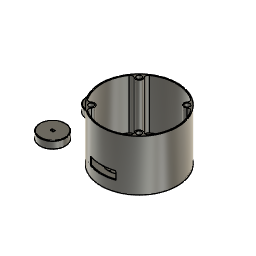
body_bottom_v4 (Autodesk Fusion 360 design; units mm, degrees)
part number: 2025-04-25-05-00-27-819
part number: 2025-04-25-05-02-16-760
part number: 2025-04-28-13-24-04-349
part number: 2025-04-28-13-40-47-946
Autodesk Fusion 360 part; units mm, degrees
sketch "Sketch1" plane through (0, 0, 0) normal (0, 0, 1) x (1, 0, 0) in component "Bottom"
  circle A0 centre (0, 0) radius 75
  dimension "d2" = 150
  constraint coincident A0.centre origin
  measures "d2" diameter of A0
extrude "Extrude1" add sketch "Sketch1" along normal blind 100 makes body 1 in component "Bottom"
shell "Shell1" thickness 2 removed faces 1 at (18.6055, 20.7304, 100) on bodies 1 in component "Bottom"
sketch "Sketch3" plane through (0, 0, 2) normal (0, 0, 1) x (-1, 0, 0) in component "Bottom"
  circle A0 centre (0, 0) radius 73
  circle A1 centre (-67, 0) radius 7
  circle A2 centre (0, 67) radius 7
  circle A3 centre (0, -67) radius 7
  circle A4 centre (67, 0) radius 7
  dimension "d11" = 14
  dimension "d12" = 14
  dimension "d13" = 14
  dimension "d14" = 14
  measures "d11" diameter of A1
  measures "d12" diameter of A2
  measures "d13" diameter of A3
  measures "d14" diameter of A4
extrude "Extrude5" add sketch "Sketch3" along normal blind 98 contours A0 A4 | A0 A2 | A0 A3 | A0 A1 picked at (69.9447, 2.5011) picked at (-0.1343, 68.6633) picked at (-0.1343, -68.6633) picked at (-68.6595, 0) bodies 1 in component "Bottom"
fillet "Fillet1" radius 6 8 edges at (72.903, 3.7623, 51) (72.903, -3.7623, 51) (-3.7623, 72.903, 51) (3.7623, 72.903, 51) (-72.903, -3.7623, 51) (3.7623, -72.903, 51) (-3.7623, -72.903, 51) (-72.903, 3.7623, 51) on bodies 1 in component "Bottom"
sketch "Sketch6" plane through (0, 0, 100) normal (0, 0, 1) x (-1, 0, 0) in component "Bottom"
  arc A0 (71.6259, 14.0974) -> (14.0974, 71.6259) centre (0, 0) ccw
  arc A1 (66.3209, 6.967) -> (71.6259, 14.0974) centre (65.7388, 12.9387) ccw
  arc A2 (66.3209, 6.967) -> (66.3209, -6.967) centre (67, 0) ccw
  arc A3 (71.6259, -14.0974) -> (66.3209, -6.967) centre (65.7388, -12.9387) ccw
  arc A4 (14.0974, -71.6259) -> (71.6259, -14.0974) centre (0, 0) ccw
  arc A5 (6.967, -66.3209) -> (14.0974, -71.6259) centre (12.9387, -65.7388) ccw
  arc A6 (6.967, -66.3209) -> (-6.967, -66.3209) centre (0, -67) ccw
  arc A7 (-14.0974, -71.6259) -> (-6.967, -66.3209) centre (-12.9387, -65.7388) ccw
  arc A8 (-71.6259, -14.0974) -> (-14.0974, -71.6259) centre (0, 0) ccw
  arc A9 (-66.3209, -6.967) -> (-71.6259, -14.0974) centre (-65.7388, -12.9387) ccw
  arc A10 (-66.3209, -6.967) -> (-66.3209, 6.967) centre (-67, 0) ccw
  arc A11 (-71.6259, 14.0974) -> (-66.3209, 6.967) centre (-65.7388, 12.9387) ccw
  arc A12 (-14.0974, 71.6259) -> (-71.6259, 14.0974) centre (0, 0) ccw
  arc A13 (-6.967, 66.3209) -> (-14.0974, 71.6259) centre (-12.9387, 65.7388) ccw
  arc A14 (-6.967, 66.3209) -> (6.967, 66.3209) centre (0, 67) ccw
  arc A15 (14.0974, 71.6259) -> (6.967, 66.3209) centre (12.9387, 65.7388) ccw
  circle A16 centre (0, 0) radius 75
  circle A17 centre (-67, 0) radius 5
  circle A18 centre (0, 67) radius 5
  circle A19 centre (67, 0) radius 5
  circle A20 centre (0, -67) radius 5
  dimension "d26" = 10
  dimension "d27" = 10
  dimension "d28" = 10
  dimension "d29" = 10
  constraint concentric A10 A17
  constraint concentric A14 A18
  constraint concentric A2 A19
  constraint concentric A6 A20
  measures "d26" diameter of A17
  measures "d27" diameter of A18
  measures "d28" diameter of A19
  measures "d29" diameter of A20
extrude "Extrude6" cut sketch "Sketch6" against normal blind 8 contours A17 | A18 | A19 | A20 bodies 1 in component "Bottom"
sketch "Sketch10" plane through (0, 0, 0) normal (0, 1, 0) x (1, 0, 0) in component "Bottom"
  line L0 (0, 100) -> (0, -200)
  constraint vertical L0
ref_plane "WorkPlane1" through (-53.033, 53.033, 0) normal (0.707107, -0.707107, 0) x (0, 0, 1) in component "Bottom"
sketch "Sketch3 (2)" plane through (0, 0, 2) normal (0, 0, 1) x (-1, 0, 0)
  line L0 (-11.65, 45) -> (11.65, 45) construction
  circle A0 centre (-14.35, 45) radius 2.7
  circle A1 centre (14.35, 45) radius 2.7
  line L1 (-14.35, 42.3) -> (-14.35, 19) construction
  line L2 (14.4157, 42.3008) -> (14.4157, 19.0008) construction
  circle A2 centre (-14.35, 16.3) radius 2.7
  circle A3 centre (14.4157, 16.3008) radius 2.7
  arc A4 (-40.6788, 60.6155) -> (-41.9696, 51.8224) centre (-37.3353, 55.6334) ccw
  arc A5 (-51.8224, 41.9696) -> (-41.9696, 51.8224) centre (-47.3762, 47.3762) ccw
  arc A6 (-51.8224, 41.9696) -> (-60.6155, 40.6788) centre (-55.6334, 37.3353) ccw
  arc A7 (-60.6155, 40.6788) -> (-60.6155, -40.6788) centre (0, 0) ccw
  arc A8 (-60.6155, -40.6788) -> (-51.8224, -41.9696) centre (-55.6334, -37.3353) ccw
  arc A9 (-41.9696, -51.8224) -> (-51.8224, -41.9696) centre (-47.3762, -47.3762) ccw
  arc A10 (-41.9696, -51.8224) -> (-40.6788, -60.6155) centre (-37.3353, -55.6334) ccw
  arc A11 (-40.6788, -60.6155) -> (40.6788, -60.6155) centre (0, 0) ccw
  arc A12 (40.6788, -60.6155) -> (41.9696, -51.8224) centre (37.3353, -55.6334) ccw
  arc A13 (51.8224, -41.9696) -> (41.9696, -51.8224) centre (47.3762, -47.3762) ccw
  arc A14 (51.8224, -41.9696) -> (60.6155, -40.6788) centre (55.6334, -37.3353) ccw
  arc A15 (60.6155, -40.6788) -> (60.6155, 40.6788) centre (0, 0) ccw
  arc A16 (60.6155, 40.6788) -> (51.8224, 41.9696) centre (55.6334, 37.3353) ccw
  arc A17 (41.9696, 51.8224) -> (51.8224, 41.9696) centre (47.3762, 47.3762) ccw
  arc A18 (41.9696, 51.8224) -> (40.6788, 60.6155) centre (37.3353, 55.6334) ccw
  arc A19 (40.6788, 60.6155) -> (-40.6788, 60.6155) centre (0, 0) ccw
  dimension "d49" = 23.3
  dimension "d50" = 5.4
  dimension "d51" = 5.4
  dimension "d52" = 23.3
  dimension "d53" = 23.3
  dimension "d54" = 5.4
  dimension "d55" = 5.4
  constraint coincident L0.start A0
  constraint coincident L0.end A1
  constraint coincident A0 L1.start
  constraint coincident A1 L2.start
  constraint coincident L1.end A2
  constraint coincident L2.end A3
  measures "d49" distance of L0.start L0.end
  measures "d50" diameter of A0
  measures "d51" diameter of A1
  measures "d52" distance of L1.start L1.end
  measures "d53" distance of L2.start L2.end
  measures "d54" diameter of A2
  measures "d55" diameter of A3
extrude "Extrude10" cut sketch "Sketch3 (2)" against normal blind 2 contours A0 | A1 | A2 | A3 sketch seen with x (-0.707107, -0.707107, 0) y (0.707107, -0.707107, 0) z (0, 0, 1) at (0, 0, 0) bodies 1 in component "Bottom"
sketch "Sketch4" plane through (0, 0, 2) normal (0, 0, 1) x (-1, 0, 0)
  circle A0 centre (-14.35, 45) radius 2.7
  circle A1 centre (-14.35, 16.3) radius 2.7
  circle A2 centre (14.35, 45) radius 2.7
  circle A3 centre (14.4157, 16.3008) radius 2.7
  arc A4 (-40.6788, 60.6155) -> (-41.9696, 51.8224) centre (-37.3353, 55.6334) ccw
  arc A5 (-51.8224, 41.9696) -> (-41.9696, 51.8224) centre (-47.3762, 47.3762) ccw
  arc A6 (-51.8224, 41.9696) -> (-60.6155, 40.6788) centre (-55.6334, 37.3353) ccw
  arc A7 (-60.6155, 40.6788) -> (-60.6155, -40.6788) centre (0, 0) ccw
  arc A8 (-60.6155, -40.6788) -> (-51.8224, -41.9696) centre (-55.6334, -37.3353) ccw
  arc A9 (-41.9696, -51.8224) -> (-51.8224, -41.9696) centre (-47.3762, -47.3762) ccw
  arc A10 (-41.9696, -51.8224) -> (-40.6788, -60.6155) centre (-37.3353, -55.6334) ccw
  arc A11 (-40.6788, -60.6155) -> (40.6788, -60.6155) centre (0, 0) ccw
  arc A12 (40.6788, -60.6155) -> (41.9696, -51.8224) centre (37.3353, -55.6334) ccw
  arc A13 (51.8224, -41.9696) -> (41.9696, -51.8224) centre (47.3762, -47.3762) ccw
  arc A14 (51.8224, -41.9696) -> (60.6155, -40.6788) centre (55.6334, -37.3353) ccw
  arc A15 (60.6155, -40.6788) -> (60.6155, 40.6788) centre (0, 0) ccw
  arc A16 (60.6155, 40.6788) -> (51.8224, 41.9696) centre (55.6334, 37.3353) ccw
  arc A17 (41.9696, 51.8224) -> (51.8224, 41.9696) centre (47.3762, 47.3762) ccw
  arc A18 (41.9696, 51.8224) -> (40.6788, 60.6155) centre (37.3353, 55.6334) ccw
  arc A19 (40.6788, 60.6155) -> (-40.6788, 60.6155) centre (0, 0) ccw
  line L0 (-42.4264, 42.4264) -> (42.4264, 42.4264) construction
  line L1 (42.4264, 42.4264) -> (42.4264, -12.5736) construction
  line L2 (42.4264, -12.5736) -> (-42.4264, -12.5736) construction
  line L3 (-42.4264, -12.5736) -> (-42.4264, 42.4264) construction
  line L4 (0, -12.5736) -> (0, -73) construction
  line L5 (-40.3762, -47.3762) -> (40.3762, -47.3762) construction
  line L6 (-42.4264, 42.4264) -> (-30.4264, 42.4264)
  line L7 (-30.4264, 42.4264) -> (-30.4264, 46.4264)
  line L8 (-30.4264, 46.4264) -> (-42.4264, 46.4264)
  line L9 (-42.4264, 46.4264) -> (-42.4264, 42.4264)
  line L10 (-42.4264, 42.4264) -> (-46.4264, 42.4264)
  line L11 (-46.4264, 42.4264) -> (-46.4264, 30.4264)
  line L12 (-46.4264, 30.4264) -> (-42.4264, 30.4264)
  line L13 (-42.4264, 30.4264) -> (-42.4264, 42.4264)
  line L14 (42.4264, 42.4264) -> (30.4264, 42.4264)
  line L15 (30.4264, 42.4264) -> (30.4264, 46.4264)
  line L16 (30.4264, 46.4264) -> (42.4264, 46.4264)
  line L17 (42.4264, 46.4264) -> (42.4264, 42.4264)
  line L18 (42.4264, 42.4264) -> (46.4264, 42.4264)
  line L19 (46.4264, 42.4264) -> (46.4264, 30.4264)
  line L20 (46.4264, 30.4264) -> (42.4264, 30.4264)
  line L21 (42.4264, 30.4264) -> (42.4264, 42.4264)
  line L22 (0, 42.4264) -> (0, -14.5736) construction
  line L23 (-42.4264, -12.5736) -> (0, -12.5736) construction
  line L24 (0, -12.5736) -> (0, -14.5736) construction
  line L25 (0, -14.5736) -> (-42.4264, -14.5736) construction
  line L26 (-42.4264, -14.5736) -> (-42.4264, -12.5736) construction
  line L27 (-30, -65) -> (30, -65) construction
  line L28 (30, -65) -> (30, -25) construction
  line L29 (30, -25) -> (-30, -25) construction
  line L30 (-30, -25) -> (-30, -65) construction
  line L31 (-30, -18) -> (30, -18)
  line L32 (30, -18) -> (30, -22)
  line L33 (30, -22) -> (-30, -22)
  line L34 (-30, -22) -> (-30, -18)
  arc A20 (30.4264, 46.4264) -> (-30.4264, 46.4264) centre (0, 19.1115) ccw
  dimension "d58" = 55
  dimension "d59" = 12
  dimension "d60" = 4
  dimension "d61" = 4
  dimension "d62" = 12
  dimension "d63" = 12
  dimension "d64" = 4
  dimension "d65" = 4
  dimension "d66" = 12
  dimension "d67" = 57
  constraint horizontal L0
  constraint vertical L1
  constraint horizontal L2
  constraint vertical L3
  constraint midpoint A5 L0.start
  constraint midpoint L2 L4.start
  constraint midpoint A11 L4.end
  constraint coincident A9 L5.start
  constraint coincident A13 L5.end
  constraint horizontal L5
  constraint horizontal L6
  constraint vertical L7
  constraint horizontal L8
  constraint vertical L9
  constraint horizontal L10
  constraint vertical L11
  constraint horizontal L12
  constraint vertical L13
  constraint horizontal L14
  constraint vertical L15
  constraint horizontal L16
  constraint vertical L17
  constraint horizontal L18
  constraint vertical L19
  constraint horizontal L20
  constraint vertical L21
  constraint midpoint L0 L22.start
  constraint perpendicular L2 L22
  constraint horizontal L23
  constraint vertical L24
  constraint horizontal L25
  constraint vertical L26
  constraint horizontal L27
  constraint vertical L28
  constraint horizontal L29
  constraint vertical L30
  constraint horizontal L31
  constraint vertical L32
  constraint horizontal L33
  constraint vertical L34
  measures "d58" distance of L0.start L2.end
  measures "d59" distance of L0.start L6.end
  measures "d60" distance of L0.start L8.end
  measures "d61" distance of L0.start L10.end
  measures "d62" distance of L0.start L12.end
  measures "d63" distance of L0.end L14.end
  measures "d64" distance of L0.end L16.end
  measures "d65" distance of L0.end L18.end
  measures "d66" distance of L0.end L20.end
  measures "d67" distance of L22.start L22.end
extrude "Extrude11" add sketch "Sketch4" along normal blind 16 contours A4 A5 A17 A18 A19 L8 L16 A20 | A5 L6 L7 L8 | A5 L11 L12 L13 | A17 L14 L15 L16 | A17 L19 L20 L21 | L31 L32 L33 L34 sketch seen with x (-0.707107, -0.707107, 0) y (0.707107, -0.707107, 0) z (0, 0, 1) at (0, 0, 0) bodies 1 in component "Bottom"
fillet "Fillet5" radius 2 2 edges at (-61.4245, -4.2324, 10) (4.2324, 61.4245, 10) on bodies 1 in component "Bottom"
sketch "Sketch5" plane through (0, -75, 0) normal (0, 1, 0) x (0, 0, 1)
  line L0 (0, 0) -> (20, 0) construction
  line L1 (20, 0) -> (36, 0) construction
  line L2 (36, 0) -> (36, -25) construction
  line L3 (36, -25) -> (20, -25)
  line L4 (20, -25) -> (20, 25)
  line L5 (20, 25) -> (36, 25)
  line L6 (36, 25) -> (36, -25)
  dimension "d74" = 20
  dimension "d75" = 16
  dimension "d76" = 25
  dimension "d77" = 50
  constraint coincident L0.start origin
  constraint horizontal L0
  constraint parallel L0 L1
  constraint perpendicular L1 L2
  constraint horizontal L3
  constraint vertical L4
  constraint horizontal L5
  constraint vertical L6
  measures "d74" distance of L0.start L0.end
  measures "d75" distance of L0.end L1.end
  measures "d76" distance of L1.end L2.end
  measures "d77" distance of L2.end L5.end
extrude "Extrude12" cut sketch "Sketch5" along normal blind 10 sketch seen with x (-0.707107, -0.707107, 0) y (0.707107, -0.707107, 0) z (0, 0, 1) at (0, 0, 0) bodies 1 in component "Bottom"
fillet "Fillet6" radius 2 2 edges at (-66.9264, 31.571, 36) (-31.571, 66.9264, 36) on bodies 1 in component "Bottom"
sketch "Sketch6 (2)" plane through (0, 0, 20) normal (0, 0, 1) x (-1, 0, 0)
  arc A0 (25, 68.5857) -> (-25, 68.5857) centre (0, 0) ccw
  line L0 (25, 68.5857) -> (25, 70.7107)
  arc A1 (25, 70.7107) -> (-25, 70.7107) centre (0, 0) ccw
  line L1 (-25, 70.7107) -> (-25, 68.5857)
  line L2 (-25, 68.5857) -> (25, 68.5857) construction
  line L3 (-25, 68.5857) -> (-25, 38.5857) construction
  line L4 (25, 68.5857) -> (25, 38.5857) construction
  line L5 (0, 68.5857) -> (0, 48.5857) construction
  dimension "d82" = 30
  dimension "d83" = 30
  dimension "d84" = 20
  constraint coincident A0.end L1.end
  constraint coincident A0.start L0.start
  constraint perpendicular L2 L3
  constraint perpendicular L2 L4
  constraint midpoint L2 L5.start
  constraint perpendicular L2 L5
  measures "d82" distance of A0.end L3.end
  measures "d83" distance of A0.start L4.end
  measures "d84" distance of L5.start L5.end
sketch "Sketch7" plane through (0, 0, 2) normal (0, 0, 1) x (-1, 0, 0)
  arc A0 (48.193, 40.424) -> (46.4264, 38.4376) centre (48.4264, 38.4376) ccw
  line L0 (46.4264, 38.4376) -> (46.4264, 30.4264)
  line L1 (42.4264, 30.4264) -> (42.4264, 42.4264)
  line L2 (42.4264, 42.4264) -> (30.4264, 42.4264)
  line L3 (30.4264, 42.4264) -> (30.4264, 46.4264)
  line L4 (-30.4264, 46.4264) -> (-30.4264, 42.4264)
  line L5 (-30.4264, 42.4264) -> (-42.4264, 42.4264)
  line L6 (-42.4264, 42.4264) -> (-42.4264, 30.4264)
  line L7 (-46.4264, 30.4264) -> (-46.4264, 38.4376)
  arc A1 (-46.4264, 38.4376) -> (-48.193, 40.424) centre (-48.4264, 38.4376) ccw
  arc A2 (-51.8224, 41.9696) -> (-48.193, 40.424) centre (-47.3762, 47.3762) ccw
  arc A3 (-51.8224, 41.9696) -> (-60.6155, 40.6788) centre (-55.6334, 37.3353) ccw
  arc A4 (-60.6155, 40.6788) -> (-60.6155, -40.6788) centre (0, 0) ccw
  arc A5 (-60.6155, -40.6788) -> (-51.8224, -41.9696) centre (-55.6334, -37.3353) ccw
  arc A6 (-41.9696, -51.8224) -> (-51.8224, -41.9696) centre (-47.3762, -47.3762) ccw
  arc A7 (-41.9696, -51.8224) -> (-40.6788, -60.6155) centre (-37.3353, -55.6334) ccw
  arc A8 (-40.6788, -60.6155) -> (40.6788, -60.6155) centre (0, 0) ccw
  arc A9 (40.6788, -60.6155) -> (41.9696, -51.8224) centre (37.3353, -55.6334) ccw
  arc A10 (51.8224, -41.9696) -> (41.9696, -51.8224) centre (47.3762, -47.3762) ccw
  arc A11 (51.8224, -41.9696) -> (60.6155, -40.6788) centre (55.6334, -37.3353) ccw
  arc A12 (60.6155, -40.6788) -> (60.6155, 40.6788) centre (0, 0) ccw
  arc A13 (60.6155, 40.6788) -> (51.8224, 41.9696) centre (55.6334, 37.3353) ccw
  arc A14 (48.193, 40.424) -> (51.8224, 41.9696) centre (47.3762, 47.3762) ccw
  circle A15 centre (-14.35, 45) radius 2.7
  circle A16 centre (-14.35, 16.3) radius 2.7
  circle A17 centre (14.35, 45) radius 2.7
  circle A18 centre (14.4157, 16.3008) radius 2.7
  line L8 (-30, -18) -> (30, -18)
  line L9 (30, -22) -> (-30, -22)
  arc A19 (30.4264, 46.4264) -> (-30.4264, 46.4264) centre (0, 19.1115) ccw
  line L10 (-30, -22) -> (-30, -18)
  line L11 (30, -18) -> (30, -22)
  line L12 (46.4264, 30.4264) -> (42.4264, 30.4264)
  line L13 (-42.4264, 30.4264) -> (-46.4264, 30.4264)
sketch "Sketch1 (2)" plane through (0, 0, 2) normal (0, 0, 1) x (-1, 0, 0) in component "Wheel"
  arc A0 (48.193, 40.424) -> (46.4264, 38.4376) centre (48.4264, 38.4376) ccw
  line L0 (46.4264, 38.4376) -> (46.4264, 30.4264)
  line L1 (42.4264, 30.4264) -> (42.4264, 42.4264)
  line L2 (42.4264, 42.4264) -> (30.4264, 42.4264)
  line L3 (30.4264, 42.4264) -> (30.4264, 46.4264)
  line L4 (-30.4264, 46.4264) -> (-30.4264, 42.4264)
  line L5 (-30.4264, 42.4264) -> (-42.4264, 42.4264)
  line L6 (-42.4264, 42.4264) -> (-42.4264, 30.4264)
  line L7 (-46.4264, 30.4264) -> (-46.4264, 38.4376)
  arc A1 (-46.4264, 38.4376) -> (-48.193, 40.424) centre (-48.4264, 38.4376) ccw
  arc A2 (-51.8224, 41.9696) -> (-48.193, 40.424) centre (-47.3762, 47.3762) ccw
  arc A3 (-51.8224, 41.9696) -> (-60.6155, 40.6788) centre (-55.6334, 37.3353) ccw
  arc A4 (-60.6155, 40.6788) -> (-60.6155, -40.6788) centre (0, 0) ccw
  arc A5 (-60.6155, -40.6788) -> (-51.8224, -41.9696) centre (-55.6334, -37.3353) ccw
  arc A6 (-41.9696, -51.8224) -> (-51.8224, -41.9696) centre (-47.3762, -47.3762) ccw
  arc A7 (-41.9696, -51.8224) -> (-40.6788, -60.6155) centre (-37.3353, -55.6334) ccw
  arc A8 (-40.6788, -60.6155) -> (40.6788, -60.6155) centre (0, 0) ccw
  arc A9 (40.6788, -60.6155) -> (41.9696, -51.8224) centre (37.3353, -55.6334) ccw
  arc A10 (51.8224, -41.9696) -> (41.9696, -51.8224) centre (47.3762, -47.3762) ccw
  arc A11 (51.8224, -41.9696) -> (60.6155, -40.6788) centre (55.6334, -37.3353) ccw
  arc A12 (60.6155, -40.6788) -> (60.6155, 40.6788) centre (0, 0) ccw
  arc A13 (60.6155, 40.6788) -> (51.8224, 41.9696) centre (55.6334, 37.3353) ccw
  arc A14 (48.193, 40.424) -> (51.8224, 41.9696) centre (47.3762, 47.3762) ccw
  circle A15 centre (-14.35, 45) radius 2.7
  circle A16 centre (-14.35, 16.3) radius 2.7
  circle A17 centre (14.35, 45) radius 2.7
  circle A18 centre (14.4157, 16.3008) radius 2.7
  line L8 (-30, -18) -> (30, -18)
  line L9 (30, -22) -> (-30, -22)
  circle A19 centre (175, 0) radius 25
  arc A20 (30.4264, 46.4264) -> (-30.4264, 46.4264) centre (0, 19.1115) ccw
  line L10 (-30, -22) -> (-30, -18)
  line L11 (30, -18) -> (30, -22)
  line L12 (46.4264, 30.4264) -> (42.4264, 30.4264)
  line L13 (-42.4264, 30.4264) -> (-46.4264, 30.4264)
  dimension "d85" = 50
  measures "d85" diameter of A19
extrude "Extrude1'" add sketch "Sketch1 (2)" along normal blind 15 separate body contours A19 makes body 2 in component "Wheel"
sketch "Sketch2" plane through (0, 0, 17) normal (0, 0, 1) x (-1, 0, 0) in component "Wheel"
  circle A0 centre (175, 0) radius 25
  line L0 (172.225, 2) -> (177.775, 2)
  line L1 (177.775, 2) -> (177.775, -2)
  line L2 (177.775, -2) -> (172.225, -2)
  line L3 (172.225, -2) -> (172.225, 2)
  line L4 (172.225, 2) -> (177.775, -2) construction
  line L5 (177.775, 2) -> (172.225, -2) construction
  point P0 (175, 0)
  dimension "d88" = 5.55
  dimension "d89" = 4
  constraint horizontal L0
  constraint perpendicular L0 L1
  constraint parallel L0 L2
  constraint parallel L1 L3
  constraint coincident L4 P0
  constraint coincident L5 P0
  constraint coincident P0 A0.centre
  measures "d88" distance of L1.end L2.end
  measures "d89" distance of L0.end L1.end
extrude "Extrude2" cut sketch "Sketch2" against normal blind 15 contours L0 L1 L2 L3 bodies 2 in component "Wheel"
fillet "Fillet1'" radius 1 2 edges at (-151.6918, 9.0404, 17) (-151.6918, 9.0404, 2) on bodies 2 in component "Wheel"
fillet "Fillet7" radius 2 6 edges at (-51.5147, 8.4853, 10) (-51.5147, -8.4853, 10) (-54.3431, -11.3137, 10) (11.3137, 54.3431, 10) (8.4853, 51.5147, 10) (-8.4853, 51.5147, 10) on bodies 1 in component "Bottom"
component "Bottom" placed x (-0.707107, 0.707107, 0) y (-0.707107, -0.707107, 0) z (0, 0, 1) at (0, 0, 0)
component "Wheel" placed x (1, 0, 0) y (0, 1, 0) z (0, 0, 1) at (0, 0, 0)
component "Wheel (1)" placed x (1, 0, 0) y (0, 1, 0) z (0, 0, 1) at (0, 0, 0)
component "Wheel" placed x (1, 0, 0) y (0, 1, 0) z (0, 0, 1) at (5.4979, 91.8311, -0.078) in component "Wheel (1)"
